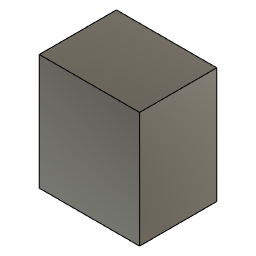
comps housing  JIRA  v1 v1 (Autodesk Fusion 360 design; units mm, degrees)
Autodesk Fusion 360 part; units mm, degrees
sketch "Esboço1" plane through (0, 0, 0) normal (0, 0, 1) x (1, 0, 0)
  line L0 (0, 0) -> (110, 0)
  line L1 (110, 0) -> (110, 140)
  line L2 (110, 140) -> (0, 140)
  line L3 (0, 140) -> (0, 0)
  dimension "d1" = 110
  dimension "d2" = 140
  constraint horizontal L0
  constraint vertical L1
  constraint horizontal L2
  constraint vertical L3
  constraint coincident L0.start L3.end
  measures "d1" distance of L0.start L0.end
  measures "d2" distance of L0.start L2.end
sketch "Esboço2" plane through (0, 0, 0) normal (0, 0, 1) x (1, 0, 0)
  line L0 (20, 180) -> (107.7649, 180)
  line L1 (107.7649, 180) -> (107.7649, 243.1748)
  line L2 (107.7649, 243.1748) -> (20, 243.1748)
  line L3 (20, 243.1748) -> (20, 180)
  constraint horizontal L0
  constraint vertical L1
  constraint horizontal L2
  constraint vertical L3
sketch "Esboço3" plane through (0, 0, 0) normal (0, 0, 1) x (1, 0, 0)
  line L0 (0, 0) -> (130, 0)
  line L1 (130, 0) -> (130, 100)
  line L2 (130, 100) -> (0, 100)
  line L3 (0, 100) -> (0, 0)
  dimension "d8" = 130
  dimension "d9" = 100
  constraint horizontal L0
  constraint vertical L1
  constraint horizontal L2
  constraint vertical L3
  constraint coincident L0.start L3.end
  measures "d8" distance of L0.start L0.end
  measures "d9" distance of L0.start L2.end
extrude "Extrusão3" add sketch "Esboço3" along normal blind 150
shell "Casca2" thickness 1.5 removed faces 0 bodies 1
